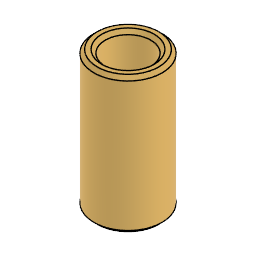
4mmIDx12mm Bushing_v1 (Autodesk Fusion 360 design; units mm, degrees)
Autodesk Fusion 360 part; units mm, degrees
sketch "Sketch1" plane through (0, 0, 0) normal (0, 0, 1) x (1, 0, 0)
  circle A0 centre (0, 0) radius 2
  circle A1 centre (0, 0) radius 3
  dimension "d1" = 4
  dimension "d2" = 6
  constraint coincident A0.centre A1.centre
  measures "d1" diameter of A0
  measures "d2" diameter of A1
extrude "Extrude1" add sketch "Sketch1" along normal blind 12
chamfer "Chamfer1" distance 0.3 angle 45 2 faces at (2.6481, -0.2484, 0) (2.6481, -0.2484, 12) tangent chain off
